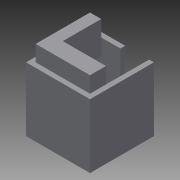
# Autodesk Inventor part: 知能ロボコン角材延長
Saved by Autodesk Inventor 2013 (Build 170138000, 138)
## iProperties
Created: 2014-06-30
Part Number: 知能ロボコン角材延長
Material: 一般
Document SubType Name: Modeling
Designer: horumo136
Density: 1 g/cm^3
Author: horumo136
Autodesk Inventor part; units mm, degrees
ref_plane "YZ Plane" through (0, 0, 0) normal (1, 0, 0) x (0, 1, 0)
ref_plane "XZ Plane" through (0, 0, 0) normal (0, 1, 0) x (-1, 0, 0)
ref_plane "XY Plane" through (0, 0, 0) normal (0, 0, 1) x (1, 0, 0)
sketch "スケッチ1" plane through (0, 0, 0) normal (0, 0, 1) x (1, 0, 0)
  line L0 (-17, 17) -> (17, 17)
  line L1 (17, 17) -> (17, -17)
  line L2 (17, -17) -> (-17, -17)
  line L3 (-17, -17) -> (-17, 17)
  line L4 (-17, 17) -> (17, -17) construction
  line L5 (17, 17) -> (-17, -17) construction
  line L6 (-20, 20) -> (20, 20)
  line L7 (20, 20) -> (20, -20)
  line L8 (20, -20) -> (-20, -20)
  line L9 (-20, -20) -> (-20, 20)
  line L10 (-20, 20) -> (20, -20) construction
  line L11 (20, 20) -> (-20, -20) construction
  point P0 (0, 0)
  dimension "d0" = 34
  dimension "d1" = 34
  dimension "d2" = 40
  dimension "d3" = 40
  constraints: 24 end point, 4 midpoint, 4 parallel, 2 horizontal, 2 perpendicular
  measures "d0" distance of L1.end L2.end
  measures "d1" distance of L0.end L1.end
  measures "d2" distance of L7.end L8.end
  measures "d3" distance of L6.end L7.end
extrude "押し出し1" add sketch "スケッチ1" along normal blind 40
sketch "スケッチ2" plane through (0, 0, 40) normal (0, 0, 1) x (1, 0, 0)
  line L0 (17, 17) -> (17, -17) projected
  line L1 (-17, -17) -> (-17, 17) projected
  line L2 (-17, -17) -> (17, -17)
  line L3 (17, -17) -> (17, -7)
  line L4 (17, -7) -> (-17, -7)
  line L5 (-17, -7) -> (-17, -17)
  line L6 (-17, 17) -> (-10, 17)
  line L7 (-10, 17) -> (-10, -7)
  line L8 (-10, -7) -> (-17, -7)
  line L9 (-17, -7) -> (-17, 17)
  point P0 (0, 0)
  dimension "d6" = 10
  dimension "d7" = 7
  constraints: 16 end point, 4 parallel, 2 horizontal, 2 perpendicular, 2 point on line
  measures "d6" distance of L3.end L2.end
  measures "d7" distance of L7.end L8.end
extrude "押し出し2" add sketch "スケッチ2" along normal blind 10 and the other way blind 10
sketch "スケッチ3" plane through (-20, 20, 0) normal (0, 1, 0) x (1, 0, 0)
  line L0 (40, -40) -> (37, -40)
  line L1 (37, -40) -> (37, -30)
  line L2 (37, -30) -> (40, -30)
  line L3 (40, -30) -> (40, -40)
  line L4 (37, -40) -> (22, -40)
  line L5 (22, -40) -> (22, -20)
  line L6 (22, -20) -> (37, -20)
  line L7 (37, -20) -> (37, -40)
  point P0 (20, 0)
  dimension "d12" = 3
  dimension "d13" = 10
  dimension "d14" = 15
  dimension "d15" = 20
  constraints: 16 end point, 4 parallel, 2 horizontal, 2 perpendicular
  measures "d12" distance of L1.end L2.end
  measures "d13" distance of L0.end L1.end
  measures "d14" distance of L5.end L6.end
  measures "d15" distance of L4.end L5.end
extrude "押し出し3" cut sketch "スケッチ3" against normal blind 10 contours L4 L5 L6 L7 L1
